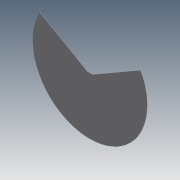
# Autodesk Inventor part: view
Saved by Autodesk Inventor 2011 (Build 150239000, 239)
## iProperties
Created: 2011-12-04
Part Number: view
Document SubType Name: Modeling
Designer: Matthew
Density: 1 g/cm^3
Author: Matthew
Autodesk Inventor part; units mm, degrees
ref_plane "YZ Plane" through (0, 0, 0) normal (1, 0, 0) x (0, 1, 0)
ref_plane "XZ Plane" through (0, 0, 0) normal (0, 1, 0) x (-1, 0, 0)
ref_plane "XY Plane" through (0, 0, 0) normal (0, 0, 1) x (1, 0, 0)
sketch "Sketch1" plane through (0, 0, 0) normal (0, 0, 1) x (1, 0, 0)
  circle A0 centre (0, 0) radius 127
  dimension "d0" = 254
  constraints: 1 centre point, 1 coincident
  measures "d0" diameter of A0
extrude "Extrusion1" add sketch "Sketch1" along normal blind 1
sketch "Sketch2" plane through (0, 0, 1) normal (0, 0, 1) x (1, 0, 0)
  circle A0 centre (0, 0) radius 127 projected
  line L0 (0.1928, 0) -> (6.5428, 0)
  line L1 (6.5428, 0) -> (-6.1572, 0)
  line L2 (-6.1572, 0) -> (-111.4922, 60.8152)
  line L3 (-6.1572, 0) -> (115.4732, 0) construction
  line L4 (6.5428, 0) -> (111.5844, 60.6458)
  line L5 (6.5428, 0) -> (127.8344, 0) construction
  dimension "d3" = 6.35
  dimension "d4" = 12.7
  dimension "d5" = 150
  dimension "d6" = 30
  constraints: 12 end point, 3 horizontal, 2 equal length, 2 point on circle, 1 collinear
  measures "d3" distance of L0.start L0.end
  measures "d4" distance of L0.end L1.end
  measures "d5" angle of L3 L2
  measures "d6" angle of L5 L4
extrude "Extrusion2" cut sketch "Sketch2" against normal blind 1 contours L4 L0 L1 L2 A0 picked at (-7.0197, 84.3704)
body "Solid1"
